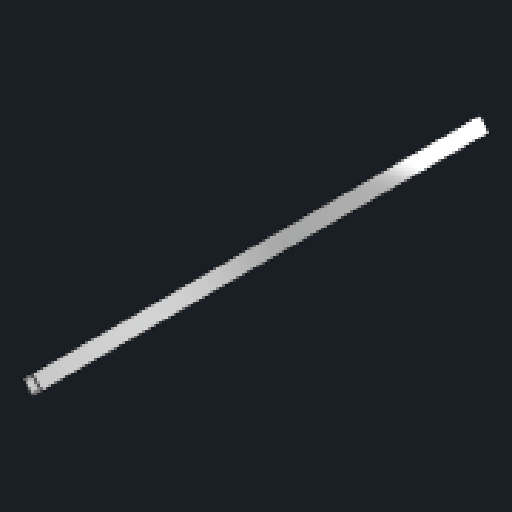
# Autodesk Inventor part: Rack Rail v3
Saved by Autodesk Inventor 2023.2 (Build 272271030, 271C)
## iProperties
Created: 2023-11-22
Part Number: Rack Rail v3
Material: Aluminum 6061
Document SubType Name: Modeling
Designer: robpl
Density: 2.7 g/cm^3
Appearance: Aluminum - Flat
Author: robpl
Autodesk Inventor part; units mm, degrees
ref_plane "YZ Plane" through (0, 0, 0) normal (1, 0, 0) x (0, 1, 0)
ref_plane "XZ Plane" through (0, 0, 0) normal (0, 1, 0) x (-1, 0, 0)
ref_plane "XY Plane" through (0, 0, 0) normal (0, 0, 1) x (1, 0, 0)
sketch "Sketch1" plane through (0, 0, 0) normal (0, 0, 1) x (1, 0, 0)
  line L0 (-2.2451, 0) -> (0, 2.2451)
  line L1 (0, 2.2451) -> (2.2451, 0)
  line L2 (2.2451, 0) -> (0, -2.2451)
  line L3 (0, -2.2451) -> (-2.2451, 0)
  line L4 (-2.2451, 0) -> (2.2451, 0) construction
  line L5 (0, 2.2451) -> (0, -2.2451) construction
  line L6 (1.6838, 0) -> (0, 1.6838)
  line L7 (0, 1.6838) -> (-1.6838, 0)
  line L8 (-1.6838, 0) -> (0, -1.6838)
  line L9 (0, -1.6838) -> (1.6838, 0)
  point P0 (0, 0)
  point P1 (0, 0)
  dimension "d4" = 3.175
  dimension "d5" = 0.3969
  constraints: 20 end point, 4 parallel, 3 perpendicular, 2 midpoint, 1 coincident, 1 horizontal, 3 other
  measures "d4" distance of L0.start L0.end
  measures "d5" distance between parallel lines of L1 L6
extrude "Extrusion2" add sketch "Sketch1" along normal blind 101
body "Solid2"
